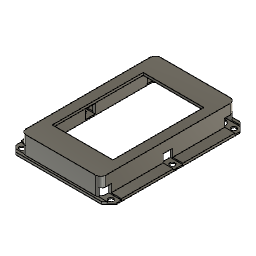
2004699A-Modified (Autodesk Fusion 360 design; units mm, degrees)
Autodesk Fusion 360 part; units mm, degrees
sketch "Sketch1" plane through (0, 0, 0) normal (0, 0, 1) x (1, 0, 0)
  line L0 (29.0445, 57.9328) -> (-12.0026, 57.9328) construction
  line L1 (41.7104, -9.3698) -> (41.7104, 10.2984) construction
  line L2 (41.7104, 10.2984) -> (41.7104, 122.9631) construction
  line L3 (29.0445, 57.9328) -> (97.0807, 57.9328) construction
  line L4 (4.7498, 120.3976) -> (4.7498, -5.9492) construction
  line L5 (79.4258, 120.3976) -> (79.4258, -5.9492) construction
  line L6 (-5.9061, 109.5756) -> (91.9438, 109.5756) construction
  line L7 (-5.9061, 6.4516) -> (90.0293, 6.4516) construction
  line L8 (6.096, 116.0526) -> (78.105, 116.0526)
  line L9 (84.201, 109.9566) -> (84.201, 6.096)
  line L10 (78.105, 0) -> (6.096, 0)
  line L11 (0, 6.096) -> (0, 109.9566)
  line L12 (6.096, 116.0526) -> (0, 109.9566)
  line L13 (78.105, 116.0526) -> (84.201, 109.9566)
  line L14 (84.201, 6.096) -> (78.105, 0)
  line L15 (6.096, 0) -> (0, 6.096)
  circle A0 centre (79.4258, 109.5756) radius 2.159
  circle A1 centre (4.7498, 109.5756) radius 2.159
  circle A2 centre (4.7498, 6.4516) radius 2.159
  circle A3 centre (79.4258, 6.4516) radius 2.159
  circle A4 centre (79.4258, 57.9328) radius 2.159
  circle A5 centre (4.7498, 57.9328) radius 2.159
  line L16 (12.9032, 114.427) -> (71.3232, 114.427)
  line L17 (75.6412, 110.109) -> (75.6412, 5.969)
  line L18 (71.3232, 1.651) -> (12.9032, 1.651)
  line L19 (8.5852, 5.969) -> (8.5852, 110.109)
  line L20 (14.9352, 112.395) -> (69.2912, 112.395)
  line L21 (73.6092, 108.077) -> (73.6092, 8.001)
  line L22 (69.2912, 3.683) -> (14.9352, 3.683)
  line L23 (10.6172, 8.001) -> (10.6172, 108.077)
  line L24 (16.7132, 96.139) -> (67.5132, 96.139)
  line L25 (67.5132, 96.139) -> (67.5132, 19.939)
  line L26 (67.5132, 19.939) -> (16.7132, 19.939)
  line L27 (16.7132, 19.939) -> (16.7132, 96.139)
  arc A6 (14.9352, 112.395) -> (10.6172, 108.077) centre (14.9352, 108.077) ccw
  arc A7 (73.6092, 108.077) -> (69.2912, 112.395) centre (69.2912, 108.077) ccw
  arc A8 (10.6172, 8.001) -> (14.9352, 3.683) centre (14.9352, 8.001) ccw
  arc A9 (69.2912, 3.683) -> (73.6092, 8.001) centre (69.2912, 8.001) ccw
  arc A10 (75.6412, 110.109) -> (71.3232, 114.427) centre (71.3232, 110.109) ccw
  arc A11 (12.9032, 114.427) -> (8.5852, 110.109) centre (12.9032, 110.109) ccw
  arc A12 (71.3232, 1.651) -> (75.6412, 5.969) centre (71.3232, 5.969) ccw
  arc A13 (8.5852, 5.969) -> (12.9032, 1.651) centre (12.9032, 5.969) ccw
  point P0 (84.201, 0)
  point P1 (0, 116.0526)
  point P2 (0, 116.0526)
  point P3 (84.201, 116.0526)
  point P4 (84.201, 0)
  point P5 (8.5852, 114.427)
  point P6 (75.6412, 114.427)
  point P7 (8.5852, 1.651)
  point P8 (10.6172, 112.395)
  point P9 (73.6092, 112.395)
  point P10 (10.6172, 3.683)
  dimension "d3" = 74.676
  dimension "d60" = 116.0526
  dimension "d61" = 84.201
  dimension "d62" = 6.096
  dimension "d63" = 6.096
  dimension "d64" = 6.096
  dimension "d65" = 6.096
  dimension "d66" = 6.096
  dimension "d67" = 6.096
  dimension "d68" = 6.096
  dimension "d69" = 6.096
  dimension "d72" = 4.318
  dimension "d73" = 4.318
  dimension "d74" = 4.318
  dimension "d75" = 4.318
  dimension "d76" = 4.318
  dimension "d77" = 4.318
  dimension "d78" = 67.056
  dimension "d79" = 112.776
  dimension "d80" = 1.6256
  dimension "d81" = 8.5598
  dimension "d82" = 108.712
  dimension "d83" = 62.992
  dimension "d84" = 2.032
  dimension "d85" = 2.032
  dimension "d86" = 76.2
  dimension "d87" = 16.256
  dimension "d88" = 50.8
  dimension "d89" = 6.096
  dimension "d98" = 4.318
  dimension "d99" = 4.318
  dimension "d100" = 4.318
  dimension "d101" = 4.318
  dimension "d102" = 4.318
  dimension "d103" = 4.318
  dimension "d104" = 4.318
  dimension "d105" = 4.318
  constraint vertical L1
  constraint horizontal L8
  constraint vertical L9
  constraint horizontal L10
  constraint vertical L11
  constraint coincident P4 P0
  constraint coincident P2 P1
  constraint coincident P2 L8
  constraint coincident P2 L11
  constraint coincident P3 L8
  constraint coincident P3 L9
  constraint coincident P4 L9
  constraint coincident P4 L10
  constraint coincident origin L10
  constraint coincident origin L11
  constraint coincident L6 A0.centre
  constraint coincident L5 A0.centre
  constraint coincident L6 A1.centre
  constraint coincident L4 A1.centre
  constraint coincident L7 A2.centre
  constraint coincident L4 A2.centre
  constraint coincident L7 A3.centre
  constraint coincident L5 A3.centre
  constraint coincident L5 A4.centre
  constraint coincident L3 A4.centre
  constraint coincident L0 A5.centre
  constraint coincident L4 A5.centre
  constraint horizontal L16
  constraint vertical L17
  constraint horizontal L18
  constraint vertical L19
  constraint horizontal L20
  constraint vertical L21
  constraint horizontal L22
  constraint vertical L23
  constraint horizontal L24
  constraint vertical L25
  constraint horizontal L26
  constraint vertical L27
  constraint coincident P8 L20
  constraint coincident P8 L23
  constraint tangent L20 A6
  constraint tangent L23 A6
  constraint coincident P9 L20
  constraint coincident P9 L21
  constraint tangent L20 A7
  constraint tangent L21 A7
  constraint coincident P10 L22
  constraint coincident P10 L23
  constraint tangent L22 A8
  constraint tangent L23 A8
  constraint tangent L21 A9
  constraint tangent L22 A9
  constraint coincident P6 L16
  constraint coincident P6 L17
  constraint tangent L16 A10
  constraint tangent L17 A10
  constraint coincident P5 L16
  constraint coincident P5 L19
  constraint tangent L16 A11
  constraint tangent L19 A11
  constraint tangent L17 A12
  constraint tangent L18 A12
  constraint coincident P7 L18
  constraint coincident P7 L19
  constraint tangent L18 A13
  constraint tangent L19 A13
  measures "d3" distance of L4 L5
  measures "d60" distance of P2 origin
  measures "d61" distance of P2 P3
  measures "d62" distance of P2 L8.start
  measures "d63" distance of P2 L11.end
  measures "d64" distance of P3 L8.end
  measures "d65" distance of P3 L9.start
  measures "d66" distance of P4 L9.end
  measures "d67" distance of P4 L10.start
  measures "d68" distance of origin L10.end
  measures "d69" distance of origin L11.start
  measures "d72" diameter of A0
  measures "d73" diameter of A1
  measures "d74" diameter of A2
  measures "d75" diameter of A3
  measures "d76" diameter of A4
  measures "d77" diameter of A5
  measures "d78" distance of P5 P6
  measures "d79" distance of P5 P7
  measures "d80" distance of L8 L16
  measures "d81" distance of L9 L17
  measures "d82" distance of P8 P10
  measures "d83" distance of P8 P9
  measures "d84" distance of L17 L21
  measures "d85" distance of L16 L20
  measures "d86" distance of L24.start L26.end
  measures "d87" distance of L22 L26
  measures "d88" distance of L25.end L26.end
  measures "d89" distance of L21 L25
  measures "d98" radius of A6
  measures "d99" radius of A7
  measures "d100" radius of A8
  measures "d101" radius of A9
  measures "d102" radius of A10
  measures "d103" radius of A11
  measures "d104" radius of A12
  measures "d105" radius of A13
sketch "Sketch2" plane through (0, 0, 0) normal (1, 0, 0) x (0, 1, 0)
  line L0 (53.8688, 1.016) -> (61.9968, 1.016)
  line L1 (61.9968, 1.016) -> (61.9968, 8.636)
  line L2 (61.9968, 8.636) -> (53.8688, 8.636)
  line L3 (53.8688, 8.636) -> (53.8688, 1.016)
  line L4 (3.8862, 0) -> (112.1664, 0)
  line L5 (6.3809, 11.5089) -> (6.3809, -11.5297) construction
  line L6 (109.6788, 11.6549) -> (109.6788, -6.3065) construction
  line L7 (105.6148, 1.016) -> (113.7428, 1.016)
  line L8 (113.7428, 1.016) -> (113.7428, 8.636)
  line L9 (113.7428, 8.636) -> (105.6148, 8.636)
  line L10 (105.6148, 8.636) -> (105.6148, 1.016)
  line L11 (109.9566, 0) -> (6.096, 0)
  line L12 (10.4449, 1.016) -> (2.3169, 1.016)
  line L13 (2.3169, 1.016) -> (2.3169, 8.636)
  line L14 (2.3169, 8.636) -> (10.4449, 8.636)
  line L15 (10.4449, 8.636) -> (10.4449, 1.016)
  point P0 (57.9328, 0)
  dimension "d46" = 7.62
  dimension "d47" = 8.128
  dimension "d48" = 4.064
  dimension "d49" = 1.016
  dimension "d106" = 7.62
  dimension "d107" = 8.128
  dimension "d108" = 1.016
  dimension "d109" = 7.62
  dimension "d110" = 8.128
  dimension "d111" = 1.016
  dimension "d112" = 4.064
  dimension "d113" = 4.064
  constraint horizontal L0
  constraint vertical L1
  constraint horizontal L2
  constraint vertical L3
  constraint perpendicular L4 L5
  constraint perpendicular L4 L6
  constraint horizontal L7
  constraint vertical L8
  constraint horizontal L9
  constraint vertical L10
  constraint horizontal L12
  constraint vertical L13
  constraint horizontal L14
  constraint vertical L15
  measures "d46" distance of L0.end L1.end
  measures "d47" distance of L1.end L2.end
  measures "d48" distance of L1 P0
  measures "d49" distance of L0.start L4
  measures "d106" distance of L7.start L9.end
  measures "d107" distance of L8.end L9.end
  measures "d108" distance of L7.start L11
  measures "d109" distance of L12.start L14.end
  measures "d110" distance of L13.end L14.end
  measures "d111" distance of L11 L12.start
  measures "d112" distance of L5 L15
  measures "d113" distance of L6 L10
extrude "Extrude6" add sketch "Sketch1" along normal blind 2.032 contours L8 L9 L10 L11 L12 L13 L14 L15
extrude "Extrude7" add sketch "Sketch1" along normal blind 17.0942 contours L16 L17 L18 L19 A10 A11 A12 A13
extrude "Extrude8" add sketch "Sketch1" along normal blind 17.0942 contours L20 L21 L22 L23 A6 A7 A8 A9
extrude "Extrude9" cut sketch "Sketch1" along normal blind 15.0622 contours L20 L21 L22 L23 A6 A7 A8 A9
extrude "Extrude10" cut sketch "Sketch2" along normal through all contours L0 L1 L2 L3
extrude "Extrude11" cut sketch "Sketch2" along normal through all contours L7 L8 L9 L10
extrude "Extrude12" cut sketch "Sketch2" along normal through all contours L12 L13 L14 L15
equation "d63 = d62"
equation "d65 = d64"
equation "d67 = d66"
equation "d69 = d68"
